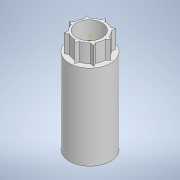
# Autodesk Inventor part: handle_base2
Saved by Autodesk Inventor 2021 (Build 250183000, 183)
## iProperties
Created: 2021-07-03
Part Number: handle_base2
Material: Generic
Document SubType Name: Modeling
Designer: teh18
Density: 1 g/cm^3
Appearance: Default
Author: teh18
Autodesk Inventor part; units mm, degrees
ref_plane "YZ Plane" through (0, 0, 0) normal (1, 0, 0) x (0, 1, 0)
ref_plane "XZ Plane" through (0, 0, 0) normal (0, 1, 0) x (-1, 0, 0)
ref_plane "XY Plane" through (0, 0, 0) normal (0, 0, 1) x (1, 0, 0)
sketch "Sketch5" plane through (0, 0, 0) normal (0, 1, 0) x (-1, 0, 0)
  line L0 (-4.3958, -5.8965) -> (-2.9002, -5.2525) projected
  arc A0 (-2.9002, -5.2525) -> (0.0521, -5.9998) centre (0, 0) ccw projected
  line L1 (0.0521, -5.9998) -> (1.0612, -7.2777) projected
  line L2 (1.0612, -7.2777) -> (1.6634, -5.7648) projected
  arc A1 (1.6634, -5.7648) -> (4.2793, -4.2057) centre (0, 0) ccw projected
  line L3 (4.2793, -4.2057) -> (5.8965, -4.3958) projected
  line L4 (5.8965, -4.3958) -> (5.2525, -2.9002) projected
  arc A2 (5.2525, -2.9002) -> (5.9998, 0.0521) centre (0, 0) ccw projected
  line L5 (5.9998, 0.0521) -> (7.2777, 1.0612) projected
  line L6 (7.2777, 1.0612) -> (5.7648, 1.6634) projected
  arc A3 (5.7648, 1.6634) -> (4.2057, 4.2793) centre (0, 0) ccw projected
  line L7 (4.2057, 4.2793) -> (4.3958, 5.8965) projected
  line L8 (4.3958, 5.8965) -> (2.9002, 5.2525) projected
  arc A4 (2.9002, 5.2525) -> (-0.0521, 5.9998) centre (0, 0) ccw projected
  line L9 (-0.0521, 5.9998) -> (-1.0612, 7.2777) projected
  line L10 (-1.0612, 7.2777) -> (-1.6634, 5.7648) projected
  arc A5 (-1.6634, 5.7648) -> (-4.2793, 4.2057) centre (0, 0) ccw projected
  line L11 (-4.2793, 4.2057) -> (-5.8965, 4.3958) projected
  line L12 (-5.8965, 4.3958) -> (-5.2525, 2.9002) projected
  arc A6 (-5.2525, 2.9002) -> (-5.9998, -0.0521) centre (0, 0) ccw projected
  line L13 (-5.9998, -0.0521) -> (-7.2777, -1.0612) projected
  line L14 (-7.2777, -1.0612) -> (-5.7648, -1.6634) projected
  arc A7 (-5.7648, -1.6634) -> (-4.2057, -4.2793) centre (0, 0) ccw projected
  line L15 (-4.2057, -4.2793) -> (-4.3958, -5.8965) projected
  circle A8 centre (0, 0) radius 29.25 projected
  arc A9 (2.8945, 5.1412) -> (-0.1, 5.8992) centre (0, 0) ccw
  line L16 (2.8945, 5.1412) -> (4.2762, 5.7362)
  line L17 (4.2762, 5.7362) -> (4.1006, 4.2421)
  arc A10 (5.6821, 1.5887) -> (4.1006, 4.2421) centre (0, 0) ccw
  line L18 (5.6821, 1.5887) -> (7.0798, 1.0323)
  line L19 (7.0798, 1.0323) -> (5.8992, 0.1)
  arc A11 (5.1412, -2.8945) -> (5.8992, 0.1) centre (0, 0) ccw
  line L20 (5.1412, -2.8945) -> (5.7362, -4.2762)
  line L21 (5.7362, -4.2762) -> (4.2421, -4.1006)
  arc A12 (1.5887, -5.6821) -> (4.2421, -4.1006) centre (0, 0) ccw
  line L22 (1.5887, -5.6821) -> (1.0323, -7.0798)
  line L23 (1.0323, -7.0798) -> (0.1, -5.8992)
  arc A13 (-2.8945, -5.1412) -> (0.1, -5.8992) centre (0, 0) ccw
  line L24 (-2.8945, -5.1412) -> (-4.2762, -5.7362)
  line L25 (-4.2762, -5.7362) -> (-4.1006, -4.2421)
  arc A14 (-5.6821, -1.5887) -> (-4.1006, -4.2421) centre (0, 0) ccw
  line L26 (-5.6821, -1.5887) -> (-7.0798, -1.0323)
  line L27 (-7.0798, -1.0323) -> (-5.8992, -0.1)
  arc A15 (-5.1412, 2.8945) -> (-5.8992, -0.1) centre (0, 0) ccw
  line L28 (-5.1412, 2.8945) -> (-5.7362, 4.2762)
  line L29 (-5.7362, 4.2762) -> (-4.2421, 4.1006)
  arc A16 (-1.5887, 5.6821) -> (-4.2421, 4.1006) centre (0, 0) ccw
  line L30 (-1.5887, 5.6821) -> (-1.0323, 7.0798)
  line L31 (-1.0323, 7.0798) -> (-0.1, 5.8992)
  circle A17 centre (0, 0) radius 4 projected
  dimension "d23" = 0.1
  constraints: 32 end point, 16 point on circle, 8 centre point, 23 other
  measures "d23" radial gap between concentric circles of A4 A9
extrude "Extrusion4" add sketch "Sketch5" along normal blind 2 and the other way blind 5 contours L16 L17 A10 L18 L19 A11 L20 L21 A12 L22 L23 A13 L24 L25 A14 L26 L27 A15 L28 L29 A16 L30 L31 A9
sketch "Sketch6" plane through (0, -5, 0) normal (0, -1, 0) x (1, 0, 0)
  line L0 (4.3958, -5.8965) -> (2.9002, -5.2525) projected
  arc A0 (-0.0521, -5.9998) -> (2.9002, -5.2525) centre (0, 0) ccw projected
  line L1 (-0.0521, -5.9998) -> (-1.0612, -7.2777) projected
  line L2 (-1.0612, -7.2777) -> (-1.6634, -5.7648) projected
  arc A1 (-4.2793, -4.2057) -> (-1.6634, -5.7648) centre (0, 0) ccw projected
  line L3 (-4.2793, -4.2057) -> (-5.8965, -4.3958) projected
  line L4 (-5.8965, -4.3958) -> (-5.2525, -2.9002) projected
  arc A2 (-5.9998, 0.0521) -> (-5.2525, -2.9002) centre (0, 0) ccw projected
  line L5 (-5.9998, 0.0521) -> (-7.2777, 1.0612) projected
  line L6 (-7.2777, 1.0612) -> (-5.7648, 1.6634) projected
  arc A3 (-4.2057, 4.2793) -> (-5.7648, 1.6634) centre (0, 0) ccw projected
  line L7 (-4.2057, 4.2793) -> (-4.3958, 5.8965) projected
  line L8 (-4.3958, 5.8965) -> (-2.9002, 5.2525) projected
  arc A4 (0.0521, 5.9998) -> (-2.9002, 5.2525) centre (0, 0) ccw projected
  line L9 (0.0521, 5.9998) -> (1.0612, 7.2777) projected
  line L10 (1.0612, 7.2777) -> (1.6634, 5.7648) projected
  arc A5 (4.2793, 4.2057) -> (1.6634, 5.7648) centre (0, 0) ccw projected
  line L11 (4.2793, 4.2057) -> (5.8965, 4.3958) projected
  line L12 (5.8965, 4.3958) -> (5.2525, 2.9002) projected
  arc A6 (5.9998, -0.0521) -> (5.2525, 2.9002) centre (0, 0) ccw projected
  line L13 (5.9998, -0.0521) -> (7.2777, -1.0612) projected
  line L14 (7.2777, -1.0612) -> (5.7648, -1.6634) projected
  arc A7 (4.2057, -4.2793) -> (5.7648, -1.6634) centre (0, 0) ccw projected
  line L15 (4.2057, -4.2793) -> (4.3958, -5.8965) projected
  circle A8 centre (0, 0) radius 29.25 projected
  circle A9 centre (0, 0) radius 20
  circle A10 centre (0, 0) radius 4 projected
  point P0 (0, 0)
  point P1 (0, 0)
  dimension "d24" = 40
  constraints: 1 centre point, 1 coincident
  measures "d24" diameter of A9
extrude "Extrusion5" add sketch "Sketch6" along normal blind 33 contours L0 A0 L1 L2 A1 L3 L4 A2 L5 L6 A3 L7 L8 A4 L9 L10 A5 L11 L12 A6 L13 L14 A7 L15 | A9
sketch "Sketch8" plane through (0, -38, 0) normal (0, -1, 0) x (0, 0, -1)
  circle A0 centre (0, 0) radius 6.1
  circle A1 centre (0, 0) radius 20 projected
  arc A2 (-5.8992, 0.1) -> (-5.1412, -2.8945) centre (0, 0) ccw projected
  line L0 (-5.8992, 0.1) -> (-7.0798, 1.0323) projected
  line L1 (-7.0798, 1.0323) -> (-5.6821, 1.5887) projected
  arc A3 (-4.1006, 4.2421) -> (-5.6821, 1.5887) centre (0, 0) ccw projected
  line L2 (-4.1006, 4.2421) -> (-4.2762, 5.7362) projected
  line L3 (-4.2762, 5.7362) -> (-2.8945, 5.1412) projected
  arc A4 (0.1, 5.8992) -> (-2.8945, 5.1412) centre (0, 0) ccw projected
  line L4 (0.1, 5.8992) -> (1.0323, 7.0798) projected
  line L5 (1.0323, 7.0798) -> (1.5887, 5.6821) projected
  arc A5 (4.2421, 4.1006) -> (1.5887, 5.6821) centre (0, 0) ccw projected
  line L6 (4.2421, 4.1006) -> (5.7362, 4.2762) projected
  line L7 (5.7362, 4.2762) -> (5.1412, 2.8945) projected
  arc A6 (5.8992, -0.1) -> (5.1412, 2.8945) centre (0, 0) ccw projected
  line L8 (5.8992, -0.1) -> (7.0798, -1.0323) projected
  line L9 (7.0798, -1.0323) -> (5.6821, -1.5887) projected
  arc A7 (4.1006, -4.2421) -> (5.6821, -1.5887) centre (0, 0) ccw projected
  line L10 (4.1006, -4.2421) -> (4.2762, -5.7362) projected
  line L11 (4.2762, -5.7362) -> (2.8945, -5.1412) projected
  arc A8 (-0.1, -5.8992) -> (2.8945, -5.1412) centre (0, 0) ccw projected
  line L12 (-0.1, -5.8992) -> (-1.0323, -7.0798) projected
  line L13 (-1.0323, -7.0798) -> (-1.5887, -5.6821) projected
  arc A9 (-4.2421, -4.1006) -> (-1.5887, -5.6821) centre (0, 0) ccw projected
  line L14 (-4.2421, -4.1006) -> (-5.7362, -4.2762) projected
  line L15 (-5.7362, -4.2762) -> (-5.1412, -2.8945) projected
  circle A10 centre (0, 0) radius 4 projected
  point P0 (0, 0)
  point P1 (1.4965, 5.9136)
  point P2 (0.2544, 6.0947)
  point P3 (5.2397, 3.1233)
  point P4 (4.4895, 4.1297)
  point P5 (5.9136, -1.4965)
  point P6 (6.0947, -0.2544)
  point P7 (3.1233, -5.2397)
  point P8 (4.1297, -4.4895)
  point P9 (-1.4965, -5.9136)
  point P10 (-0.2544, -6.0947)
  point P11 (-5.2397, -3.1233)
  point P12 (-4.4895, -4.1297)
  point P13 (-5.9136, 1.4965)
  point P14 (-6.0947, 0.2544)
  point P15 (-3.1233, 5.2397)
  point P16 (-4.1297, 4.4895)
  dimension "d19" = 12.2
  constraints: 1 centre point, 1 coincident
  measures "d19" diameter of A0
extrude "Extrusion7" cut sketch "Sketch8" against normal blind 10 contours A0 L8 A6 L7 | L7 A6 L8 A0 L9 A7 L10 L11 A8 L12 L13 A9 L14 L15 A2 L0 L1 A3 L2 L3 A4 L4 L5 A5 L6 | A0 L6 L7 | L8 L9 A0 | L6 A5 L5 A0 | A0 L10 A7 L9 | A0 L4 L5 | L10 L11 A0 | L4 A4 L3 A0 | A0 L12 A8 L11 | A0 L2 L3 | L12 L13 A0 | L2 A3 L1 A0 | A0 L14 A9 L13 | A0 L0 L1 | L14 L15 A0 | L0 A2 L15 A0 | A10
body "Solid2"
